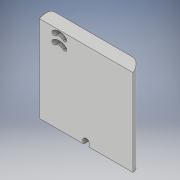
# Autodesk Inventor part: Case Back
Saved by Autodesk Inventor 2019 (Build 230136000, 136)
## iProperties
Created: 2022-04-25
Part Number: Case Back
Material: Generic
Document SubType Name: Modeling
Designer: Loxei
Density: 1 g/cm^3
Appearance: Default
Author: Loxei
Autodesk Inventor part; units mm, degrees
ref_plane "YZ Plane" through (0, 0, 0) normal (1, 0, 0) x (0, 1, 0)
ref_plane "XZ Plane" through (0, 0, 0) normal (0, 1, 0) x (-1, 0, 0)
ref_plane "XY Plane" through (0, 0, 0) normal (0, 0, 1) x (1, 0, 0)
sketch "Sketch2" plane through (0, 0, 0) normal (1, 0, 0) x (0, 1, 0)
  line L0 (43.74, 0) -> (-43.74, 0) construction
  line L1 (0, 65.172) -> (0, -65.172) construction
  spline S0 degree 3 poles (-5.8666, 35) (13.8832, 21.2522) (-10.0462, -16.0043) (8.551, -35) knots 1 1 1 1 2 2 2 2
  line L2 (-5.8666, 35) -> (13.8832, 21.2522) construction
  line L3 (13.8832, 21.2522) -> (-10.0462, -16.0043) construction
  line L4 (-10.0462, -16.0043) -> (8.551, -35) construction
  line L5 (-5.8666, 35) -> (-40.8666, 35)
  line L6 (-1.7165, 31) -> (-40.8666, 31)
  line L7 (-40.8666, 35) -> (-40.8666, 31)
  line L8 (8.551, -35) -> (-40.8666, -35)
  line L9 (-40.8666, -35) -> (-40.8666, -31)
  line L10 (-40.8666, -31) -> (5.392, -31)
  point P0 (0, 0)
  point P1 (0, 0)
  point P2 (0, 0)
  point P3 (0, 0)
  point P4 (0, 0)
  dimension "d0" = 35
  dimension "d1" = 4
  dimension "d2" = 4
  constraints: 16 end point, 4 midpoint, 4 perpendicular, 2 horizontal, 2 symmetric about line, 2 vertical, 1 coincident, 1 parallel, 5 other
  measures "d0" distance of L2.start L5.end
  measures "d1" distance between parallel lines of L5 L6
  measures "d2" distance of L8.end L9.end
extrude "Extrusion1" add sketch "Sketch2" along normal blind 50 contours S0 L8 L9 L10
fillet "Fillet1" radius 4 2 edges at (50, -16.1578, -35) (0, -16.1578, -35)
sketch "Sketch3" plane through (46, 8.551, -35) normal (0, 0, -1) x (-1, 0, 0)
  circle A0 centre (21.067, -48.0176) radius 1.875
  line L0 (42, -49.4176) -> (0, -49.4176) projected
  arc A1 (38.2925, -5.9026) -> (32.5085, -5.9701) centre (35.4376, -9.1181) ccw construction
  arc A2 (39.0228, -5.08) -> (31.7591, -5.1648) centre (35.4376, -9.1181) ccw
  arc A3 (37.5622, -6.7252) -> (33.2578, -6.7754) centre (35.4376, -9.1181) ccw
  arc A4 (37.5622, -6.7252) -> (39.0228, -5.08) centre (38.2925, -5.9026) ccw
  arc A5 (31.7591, -5.1648) -> (33.2578, -6.7754) centre (32.5085, -5.9701) ccw
  arc A6 (38.2925, -10.2026) -> (32.5085, -10.2701) centre (35.4376, -13.4181) ccw construction
  arc A7 (39.0228, -9.38) -> (31.7591, -9.4648) centre (35.4376, -13.4181) ccw
  arc A8 (37.5622, -11.0252) -> (33.2578, -11.0754) centre (35.4376, -13.4181) ccw
  arc A9 (37.5622, -11.0252) -> (39.0228, -9.38) centre (38.2925, -10.2026) ccw
  arc A10 (31.7591, -9.4648) -> (33.2578, -11.0754) centre (32.5085, -10.2701) ccw
  line L1 (35.4376, -14.6833) -> (35.4376, -1.9908) construction
  point P0 (46, -8.551)
  dimension "d6" = 3.75
  dimension "d7" = 1.4
  dimension "d10" = 4.3
  dimension "d11" = 4.3
  dimension "d12" = 3.2
  dimension "d13" = 3.2
  dimension "d14" = 4.3
  constraints: 20 point on circle, 11 centre point, 8 tangent, 2 end point, 2 point on line, 1 vertical
  measures "d6" diameter of A0
  measures "d7" distance from line of L0 A0.centre
  measures "d10" radius of A1
  measures "d11" radius of A6
  measures "d12" radius of A8
  measures "d13" radius of A3
  measures "d14" distance of A6.centre A1.centre
extrude "Extrusion2" cut sketch "Sketch3" against normal blind 4
equation "\"d11\" = d10"
equation "\"d13\" = d12"
equation "\"d14\" = d11"
body "Solid1"
